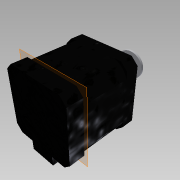
# Autodesk Inventor part: stepmotor small
Saved by Autodesk Inventor 2014 (Build 180170000, 170)
## iProperties
Created: 2015-12-16
Part Number: stepmotor small
Material: Steel
Document SubType Name: Modeling
Designer: admin
Density: 0.93 g/cm^3
Appearance: Steel
Author: admin
Autodesk Inventor part; units mm, degrees
ref_plane "YZ Plane" through (0, 0, 0) normal (1, 0, 0) x (0, 1, 0)
ref_plane "XZ Plane" through (0, 0, 0) normal (0, 1, 0) x (-1, 0, 0)
ref_plane "XY Plane" through (0, 0, 0) normal (0, 0, 1) x (1, 0, 0)
sketch "Sketch1" plane through (0, 0, 0) normal (0, 1, 0) x (-1, 0, 0)
  line L0 (-21, 21) -> (21, 21)
  line L1 (21, 21) -> (21, -21)
  line L2 (21, -21) -> (-21, -21)
  line L3 (-21, -21) -> (-21, 21)
  line L4 (-21, 21) -> (21, -21) construction
  line L5 (21, 21) -> (-21, -21) construction
  point P0 (0, 0)
  dimension "d0" = 42
  dimension "d1" = 42
  constraints: 12 end point, 2 midpoint, 2 parallel, 1 horizontal, 1 perpendicular
  measures "d0" distance of L1.end L2.end
  measures "d1" distance of L0.end L1.end
extrude "Extrusion1" add sketch "Sketch1" along normal blind 45
sketch "Sketch3" plane through (0, 45, 0) normal (0, 1, 0) x (1, 0, 0)
  circle A0 centre (0, 0) radius 10
  dimension "d4" = 20
  constraints: 1 centre point, 1 coincident
  measures "d4" diameter of A0
extrude "Extrusion2" add sketch "Sketch3" along normal blind 2
sketch "Sketch4" plane through (0, 45, 0) normal (0, 1, 0) x (1, 0, 0)
  circle A0 centre (0, 0) radius 10 projected
  line L0 (-15.5, 15.5) -> (15.5, 15.5)
  line L1 (15.5, 15.5) -> (15.5, -15.5)
  line L2 (15.5, -15.5) -> (-15.5, -15.5)
  line L3 (-15.5, -15.5) -> (-15.5, 15.5)
  line L4 (-15.5, 15.5) -> (15.5, -15.5) construction
  line L5 (15.5, 15.5) -> (-15.5, -15.5) construction
  circle A1 centre (15.5, 15.5) radius 1.5
  circle A2 centre (-15.5, 15.5) radius 1.5
  circle A3 centre (-15.5, -15.5) radius 1.5
  circle A4 centre (15.5, -15.5) radius 1.5
  dimension "d7" = 31
  dimension "d8" = 31
  dimension "d9" = 3
  dimension "d10" = 3
  dimension "d11" = 3
  dimension "d12" = 3
  constraints: 12 end point, 4 centre point, 4 coincident, 2 midpoint, 2 parallel, 1 horizontal, 1 perpendicular
  measures "d7" distance of L1.end L2.end
  measures "d8" distance of L0.end L1.end
  measures "d9" diameter of A1
  measures "d10" diameter of A2
  measures "d11" diameter of A3
  measures "d12" diameter of A4
extrude "Extrusion3" cut sketch "Sketch4" against normal blind 10 contours L3 A2 L0 | L0 A2 L3 | A1 L1 L0 | L0 L1 A1 | A3 L2 L3 | L3 L2 A3 | A4 L2 L1 | L1 L2 A4
chamfer "Chamfer1" distance 4 angle 45 4 edges at (-21, 22.5, -21) (21, 22.5, -21) (-21, 22.5, 21) (21, 22.5, 21)
sketch "Sketch5" plane through (0, 47, 0) normal (0, 1, 0) x (1, 0, 0)
  circle A0 centre (0, 0) radius 10 projected
  circle A1 centre (0, 0) radius 2.5
  dimension "d18" = 5
  constraints: 1 centre point, 1 coincident
  measures "d18" diameter of A1
extrude "Extrusion4" add sketch "Sketch5" along normal blind 21 contours A1
ref_plane "Work Plane1" through (0, 9.2, 0) normal (0, -1, 0) x (1, 0, 0)
sketch "Sketch6" plane through (0, 9.2, 0) normal (0, -1, 0) x (1, 0, 0)
  line L0 (17, 21) -> (21, 17) projected
  line L1 (17, 21) -> (-17, 21) projected
  line L2 (-21, 17) -> (-17, 21) projected
  line L3 (-21, 17) -> (-21, -17) projected
  line L4 (-17, -21) -> (-21, -17) projected
  line L5 (-17, -21) -> (17, -21) projected
  line L6 (21, -17) -> (17, -21) projected
  line L7 (21, -17) -> (21, 17) projected
  arc A0 (21, 13) -> (13, 21) centre (9.5, 9.5) ccw
  point P0 (0, 0)
  constraints: 2 point on circle, 2 point on line, 1 centre point
extrude "Extrusion5" cut sketch "Sketch6" against normal blind 28 contours L0 L7 A0 L1
pattern_circular "Circular Pattern1" count 4 over 360 about axis through (0, 47, 0) along (0, 1, 0) of "Extrusion5"
sketch "Sketch7" plane through (0, 68, 0) normal (0, 1, 0) x (1, 0, 0)
  circle A0 centre (0, 0) radius 2.5 projected
  circle A1 centre (0, 0) radius 9
  dimension "d27" = 18
  constraints: 1 centre point, 1 coincident
  measures "d27" diameter of A1
extrude "Extrusion6" add sketch "Sketch7" against normal blind 1.5 separate body
sketch "Sketch8" plane through (0, 66.5, 0) normal (0, -1, 0) x (1, 0, 0)
  circle A0 centre (0, 0) radius 2.5 projected
  circle A1 centre (0, 0) radius 9 projected
  circle A2 centre (0, 0) radius 5.5
  dimension "d30" = 11
  constraints: 1 centre point, 1 coincident
  measures "d30" diameter of A2
extrude "Extrusion7" add sketch "Sketch8" along normal blind 7.5 contours A2 bodies 2
sketch "Sketch9" plane through (0, 59, 0) normal (0, -1, 0) x (1, 0, 0)
  circle A0 centre (0, 0) radius 2.5 projected
  circle A1 centre (0, 0) radius 5.5 projected
  circle A2 centre (0, 0) radius 9
  dimension "d33" = 18
  constraints: 1 centre point, 1 coincident
  measures "d33" diameter of A2
extrude "Extrusion8" add sketch "Sketch9" along normal blind 9 contours A1 | A2 bodies 2
sketch "Sketch10" plane through (17, 0, -21) normal (0, 0, -1) x (-1, 0, 0)
  line L0 (4, 9.2) -> (0, 9.2) projected
  line L1 (34, 0) -> (0, 0) projected
  line L2 (9, 0) -> (25, 0)
  line L3 (25, 0) -> (25, 9.2)
  line L4 (25, 9.2) -> (9, 9.2)
  line L5 (9, 9.2) -> (9, 0)
  point P0 (17, 0)
  dimension "d36" = 16
  dimension "d37" = 8
  constraints: 8 end point, 2 parallel, 2 point on line, 1 horizontal, 1 perpendicular
  measures "d36" distance between parallel lines of L5 L3
  measures "d37" distance from line of point (17, 0) L5
extrude "Extrusion9" add sketch "Sketch10" along normal blind 6 bodies 1
body "Solid1"
body "Solid2"
